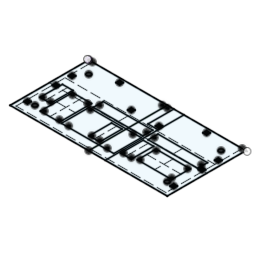
_Drill Guide.1d35a3b7-5dbf-4833-a90d-6280b39ef4eb (Autodesk Fusion 360 design; units mm, degrees)
Autodesk Fusion 360 part; units mm, degrees
sketch "Sketch1" plane through (0, 0, 0) normal (0, 1, 0) x (1, 0, 0)
  line L0 (0, 0) -> (304.8, 0) construction
  line L1 (304.8, 0) -> (304.8, -152.4) construction
  line L2 (304.8, -152.4) -> (0, -152.4) construction
  line L3 (0, -152.4) -> (0, 0) construction
  line L4 (297.775, 0) -> (297.775, -147.9) construction
  line L5 (297.775, -147.9) -> (7.025, -147.9) construction
  line L6 (7.025, -147.9) -> (7.025, 0) construction
  line L7 (39.025, -70.5) -> (76.025, -70.5)
  line L8 (76.025, -70.5) -> (76.025, -132.9)
  line L9 (76.025, -132.9) -> (39.025, -132.9)
  line L10 (39.025, -132.9) -> (39.025, -70.5)
  circle A0 centre (42.95, -74.425) radius 1.625
  line L11 (57.525, -70.5) -> (57.525, -132.9) construction
  circle A1 centre (72.1, -74.425) radius 1.625
  line L12 (39.025, -101.7) -> (76.025, -101.7) construction
  circle A2 centre (72.1, -128.975) radius 1.625
  circle A3 centre (42.95, -128.975) radius 1.625
  line L13 (15.525, -66.5) -> (35.875, -66.5)
  line L14 (35.875, -66.5) -> (35.875, -109.9)
  line L15 (35.875, -109.9) -> (15.525, -109.9)
  line L16 (15.525, -109.9) -> (15.525, -66.5)
  circle A4 centre (18.08, -107.345) radius 1.555
  line L17 (25.7, -66.5) -> (25.7, -109.9) construction
  circle A5 centre (33.32, -107.345) radius 1.555
  line L18 (80.025, -79.56) -> (181.625, -79.56)
  line L19 (181.625, -79.56) -> (181.625, -132.9)
  line L20 (181.625, -132.9) -> (80.025, -132.9)
  line L21 (80.025, -132.9) -> (80.025, -79.56)
  circle A6 centre (85.105, -82.1) radius 1.65
  circle A7 centre (91.455, -130.36) radius 1.65
  circle A8 centre (167.655, -82.1) radius 1.65
  circle A9 centre (166.385, -130.36) radius 1.65
  line L22 (7.025, -52.9) -> (297.775, -52.9) construction
  line L23 (187.625, -82) -> (207.975, -82)
  line L24 (207.975, -82) -> (207.975, -125.4)
  line L25 (207.975, -125.4) -> (187.625, -125.4)
  line L26 (187.625, -125.4) -> (187.625, -82)
  circle A10 centre (190.18, -122.845) radius 1.555
  line L27 (197.8, -82) -> (197.8, -125.4) construction
  circle A11 centre (205.42, -122.845) radius 1.555
  circle A12 centre (145.82, -124.545) radius 1.555
  circle A13 centre (130.58, -124.545) radius 1.555
  line L28 (148.375, -83.7) -> (148.375, -127.1)
  line L29 (148.375, -127.1) -> (128.025, -127.1)
  line L30 (128.025, -127.1) -> (128.025, -83.7)
  line L31 (138.2, -83.7) -> (138.2, -127.1) construction
  line L32 (128.025, -83.7) -> (148.375, -83.7)
  line L33 (215.125, -84.4) -> (281.275, -84.4)
  line L34 (281.275, -84.4) -> (281.275, -120.4)
  line L35 (281.275, -120.4) -> (215.125, -120.4)
  line L36 (215.125, -120.4) -> (215.125, -84.4)
  circle A14 centre (217.675, -86.95) radius 1.55
  line L37 (248.2, -84.4) -> (248.2, -120.4) construction
  line L38 (215.125, -102.4) -> (281.275, -102.4) construction
  circle A15 centre (278.725, -86.95) radius 1.55
  circle A16 centre (217.675, -117.85) radius 1.55
  circle A17 centre (278.725, -117.85) radius 1.55
  line L39 (84.065, -55.86) -> (180.125, -55.86)
  line L40 (180.125, -55.86) -> (180.125, -74.96)
  line L41 (180.125, -74.96) -> (84.065, -74.96)
  line L42 (84.065, -74.96) -> (84.065, -55.86)
  circle A18 centre (177.625, -65.46) radius 1.5
  line L43 (132.095, -55.86) -> (132.095, -74.96) construction
  circle A19 centre (86.565, -65.46) radius 1.5
  line L44 (191.715, -76.4) -> (191.715, -57.3)
  line L45 (239.745, -57.3) -> (239.745, -76.4) construction
  line L46 (287.775, -76.4) -> (191.715, -76.4)
  line L47 (191.715, -57.3) -> (287.775, -57.3)
  circle A20 centre (285.275, -66.9) radius 1.5
  circle A21 centre (194.215, -66.9) radius 1.5
  line L48 (287.775, -57.3) -> (287.775, -76.4)
  line L49 (7.025, -125.9) -> (14.025, -125.9)
  line L50 (14.025, -125.9) -> (14.025, -132.9)
  line L51 (14.025, -132.9) -> (7.025, -132.9)
  line L52 (7.025, -132.9) -> (7.025, -125.9)
  line L53 (7.025, -70.9) -> (14.025, -70.9)
  line L54 (14.025, -70.9) -> (14.025, -77.9)
  line L55 (14.025, -77.9) -> (7.025, -77.9)
  line L56 (7.025, -77.9) -> (7.025, -70.9)
  line L57 (7.025, -39.4) -> (14.025, -39.4)
  line L58 (14.025, -39.4) -> (14.025, -46.4)
  line L59 (14.025, -46.4) -> (7.025, -46.4)
  line L60 (7.025, -46.4) -> (7.025, -39.4)
  line L61 (122.025, -39.4) -> (129.025, -39.4)
  line L62 (129.025, -39.4) -> (129.025, -46.4)
  line L63 (129.025, -46.4) -> (122.025, -46.4)
  line L64 (122.025, -46.4) -> (122.025, -39.4)
  line L65 (152.4, 0) -> (152.4, -147.9) construction
  circle A22 centre (68.025, -8) radius 1.5
  circle A23 centre (10.525, -42.9) radius 1.5
  circle A24 centre (10.525, -74.4) radius 1.5
  circle A25 centre (10.525, -129.4) radius 1.5
  circle A26 centre (125.525, -42.9) radius 1.5
  line L66 (0, 0) -> (304.8, 0)
  line L67 (304.8, 0) -> (304.8, -152.4)
  line L68 (304.8, -152.4) -> (0, -152.4)
  line L69 (0, -152.4) -> (0, 0)
  line L70 (152.4, 0) -> (152.4, -152.4)
  line L71 (-0.1, 0) -> (-2.5, 0)
  line L72 (307.3, 0) -> (304.9, 0)
  line L73 (0, 0) -> (-0.1, 0)
  line L74 (304.9, 0) -> (304.8, 0)
  line L75 (184.625, 0) -> (184.625, -152.4)
  line L76 (165, 0) -> (165, -50)
  line L77 (165, -50) -> (184.625, -50)
  circle A27 centre (24, -128.4) radius 3.95
  line L78 (0, -76.2) -> (304.8, -76.2) construction
  circle A28 centre (24, -24) radius 3.95
  circle A29 centre (280.8, -24) radius 3.95
  circle A30 centre (280.8, -128.4) radius 3.95
  circle A31 centre (147.4, -4.75) radius 1.5
  circle A32 centre (157.4, -4.75) radius 1.5
  line L79 (64.525, -4.5) -> (71.525, -4.5)
  line L80 (71.525, -4.5) -> (71.525, -11.5)
  line L81 (71.525, -11.5) -> (64.525, -11.5)
  line L82 (64.525, -11.5) -> (64.525, -4.5)
  line L83 (233.275, -11.5) -> (240.275, -11.5)
  circle A33 centre (236.775, -8) radius 1.5
  line L84 (240.275, -11.5) -> (240.275, -4.5)
  line L85 (240.275, -4.5) -> (233.275, -4.5)
  line L86 (233.275, -4.5) -> (233.275, -11.5)
  line L87 (297.775, -39.4) -> (290.775, -39.4)
  line L88 (290.775, -39.4) -> (290.775, -46.4)
  circle A34 centre (294.275, -42.9) radius 1.5
  line L89 (290.775, -46.4) -> (297.775, -46.4)
  line L90 (297.775, -46.4) -> (297.775, -39.4)
  line L91 (297.775, -70.9) -> (290.775, -70.9)
  line L92 (290.775, -70.9) -> (290.775, -77.9)
  circle A35 centre (294.275, -74.4) radius 1.5
  line L93 (297.775, -77.9) -> (297.775, -70.9)
  line L94 (290.775, -77.9) -> (297.775, -77.9)
  line L95 (297.775, -125.9) -> (290.775, -125.9)
  line L96 (290.775, -125.9) -> (290.775, -132.9)
  circle A36 centre (294.275, -129.4) radius 1.5
  line L97 (290.775, -132.9) -> (297.775, -132.9)
  line L98 (297.775, -132.9) -> (297.775, -125.9)
  circle A37 centre (179.275, -42.9) radius 1.5
  line L99 (175.775, -46.4) -> (182.775, -46.4)
  line L100 (182.775, -46.4) -> (182.775, -39.4)
  line L101 (175.775, -39.4) -> (175.775, -46.4)
  line L102 (182.775, -39.4) -> (175.775, -39.4)
  dimension "d1" = 304.8
  dimension "d2" = 152.4
  dimension "d3" = 290.75
  dimension "d4" = 147.9
  dimension "d5" = 7.025
  dimension "d6" = 3.25
  dimension "d7" = 37
  dimension "d8" = 62.4
  dimension "d9" = 3.925
  dimension "d10" = 3.925
  dimension "d11" = 32
  dimension "d13" = 20.35
  dimension "d14" = 43.4
  dimension "d15" = 3.11
  dimension "d16" = 2.555
  dimension "d17" = 2.555
  dimension "d18" = 8.5
  dimension "d19" = 42.5
  dimension "d20" = 19.5
  dimension "d21" = 101.6
  dimension "d22" = 53.34
  dimension "d23" = 3.3
  dimension "d24" = 3.3
  dimension "d25" = 3.3
  dimension "d26" = 3.3
  dimension "d27" = 96.52
  dimension "d28" = 2.54
  dimension "d29" = 13.97
  dimension "d30" = 2.54
  dimension "d31" = 15.24
  dimension "d32" = 50.8
  dimension "d33" = 90.17
  dimension "d34" = 50.8
  dimension "d35" = 19.5
  dimension "d36" = 73
  dimension "d38" = 20.35
  dimension "d39" = 43.4
  dimension "d40" = 3.11
  dimension "d41" = 2.555
  dimension "d42" = 2.555
  dimension "d43" = 27
  dimension "d45" = 6
  dimension "d46" = 20.35
  dimension "d47" = 43.4
  dimension "d48" = 3.11
  dimension "d49" = 2.555
  dimension "d50" = 2.555
  dimension "d51" = 25.3
  dimension "d52" = 48
  dimension "d53" = 66.15
  dimension "d54" = 36
  dimension "d55" = 3.1
  dimension "d56" = 2.55
  dimension "d57" = 2.55
  dimension "d58" = 32
  dimension "d59" = 16.5
  dimension "d60" = 96.06
  dimension "d61" = 19.1
  dimension "d62" = 3
  dimension "d63" = 9.6
  dimension "d64" = 2.5
  dimension "d65" = 4.6
  dimension "d66" = 1.5
  dimension "d67" = 96.06
  dimension "d68" = 19.1
  dimension "d69" = 3
  dimension "d70" = 9.6
  dimension "d71" = 2.5
  dimension "d72" = 10
  dimension "d73" = 8
  dimension "d74" = 7
  dimension "d75" = 7
  dimension "d76" = 15
  dimension "d77" = 7
  dimension "d78" = 7
  dimension "d79" = 70
  dimension "d80" = 7
  dimension "d81" = 7
  dimension "d82" = 101.5
  dimension "d86" = 7
  dimension "d87" = 7
  dimension "d88" = 115
  dimension "d89" = 101.5
  dimension "d90" = 3
  dimension "d93" = 3
  dimension "d94" = 3.5
  dimension "d95" = 3.5
  dimension "d96" = 3
  dimension "d97" = 3.5
  dimension "d98" = 3.5
  dimension "d99" = 3
  dimension "d100" = 3.5
  dimension "d101" = 3.5
  dimension "d102" = 3
  dimension "d103" = 3.5
  dimension "d104" = 3.5
  dimension "d127" = 3
  dimension "d130" = 19.625
  dimension "d131" = 50
  dimension "d132" = 7.9
  dimension "d133" = 24
  dimension "d134" = 24
  dimension "d135" = 3
  dimension "d136" = 3
  dimension "d137" = 10
  dimension "d140" = 5
  dimension "d141" = 4.75
  dimension "d145" = 7
  dimension "d146" = 7
  dimension "d147" = 3.5
  dimension "d148" = 3.5
  dimension "d149" = 4.5
  dimension "d150" = 4.75
  dimension "d151" = 57.5
  dimension "d152" = 52.9
  constraint horizontal L0
  constraint vertical L1
  constraint horizontal L2
  constraint vertical L3
  constraint coincident L0.start L3.end
  constraint vertical L4
  constraint horizontal L5
  constraint vertical L6
  constraint coincident L0 L6.end
  constraint horizontal L7
  constraint vertical L8
  constraint horizontal L9
  constraint vertical L10
  constraint midpoint L7 L11.start
  constraint midpoint L9 L11.end
  constraint symmetric A0 L11 A1
  constraint midpoint L10 L12.start
  constraint midpoint L8 L12.end
  constraint symmetric A0 L12 A3
  constraint symmetric A1 L12 A2
  constraint horizontal L13
  constraint vertical L14
  constraint horizontal L15
  constraint vertical L16
  constraint midpoint L13 L17.start
  constraint midpoint L15 L17.end
  constraint symmetric A4 L17 A5
  constraint horizontal L18
  constraint vertical L19
  constraint horizontal L20
  constraint vertical L21
  constraint coincident L6 L22.start
  constraint coincident L4 L22.end
  constraint perpendicular L4 L22
  constraint horizontal L23
  constraint vertical L24
  constraint horizontal L25
  constraint vertical L26
  constraint midpoint L23 L27.start
  constraint midpoint L25 L27.end
  constraint symmetric A10 L27 A11
  constraint horizontal L32
  constraint vertical L28
  constraint horizontal L29
  constraint vertical L30
  constraint midpoint L31.start L32
  constraint midpoint L31.end L29
  constraint symmetric A12 A13 L31
  constraint horizontal L33
  constraint vertical L34
  constraint horizontal L35
  constraint vertical L36
  constraint midpoint L33 L37.start
  constraint midpoint L35 L37.end
  constraint midpoint L36 L38.start
  constraint midpoint L34 L38.end
  constraint symmetric A14 L37 A15
  constraint symmetric A14 L38 A16
  constraint symmetric L38 A15 A17
  constraint horizontal L39
  constraint vertical L40
  constraint horizontal L41
  constraint vertical L42
  constraint midpoint L39 L43.start
  constraint midpoint L41 L43.end
  constraint symmetric A18 L43 A19
  constraint horizontal L47
  constraint vertical L48
  constraint horizontal L46
  constraint vertical L44
  constraint midpoint L45.start L47
  constraint midpoint L45.end L46
  constraint symmetric L45 A20 A21
  constraint horizontal L49
  constraint vertical L50
  constraint horizontal L51
  constraint vertical L52
  constraint coincident L6 L49.start
  constraint horizontal L53
  constraint vertical L54
  constraint horizontal L55
  constraint vertical L56
  constraint coincident L6 L53.start
  constraint horizontal L57
  constraint vertical L58
  constraint horizontal L59
  constraint vertical L60
  constraint coincident L6 L57.start
  constraint horizontal L61
  constraint vertical L62
  constraint horizontal L63
  constraint vertical L64
  constraint midpoint L5 L65.end
  constraint horizontal L66
  constraint vertical L67
  constraint horizontal L68
  constraint vertical L69
  constraint midpoint L68 L70.end
  constraint perpendicular L1 L72
  constraint perpendicular L67 L74
  constraint coincident L66 L75.start
  constraint coincident L68 L75.end
  constraint perpendicular L68 L75
  constraint coincident L66 L76.start
  constraint perpendicular L22 L76
  constraint coincident L75 L77.end
  constraint perpendicular L75 L77
  constraint midpoint L3 L78.start
  constraint midpoint L67 L78.end
  constraint symmetric A27 L78 A28
  constraint symmetric L70 A27 A30
  constraint symmetric L70 A28 A29
  constraint horizontal L79
  constraint vertical L80
  constraint horizontal L81
  constraint vertical L82
  constraint symmetric L49.start L65 L95.start
  constraint symmetric L49.end L65 L95.end
  constraint symmetric L50.end L65 L96.end
  constraint symmetric L51.end L65 L97.end
  constraint symmetric L53.start L65 L91.start
  constraint symmetric L53.end L65 L91.end
  constraint symmetric L54.end L65 L92.end
  constraint symmetric L55.end L65 L93.start
  constraint symmetric L57.start L65 L87.start
  constraint symmetric L57.end L65 L87.end
  constraint symmetric L58.end L65 L88.end
  constraint symmetric L59.end L65 L89.end
  constraint symmetric L61.start L65 L100.end
  constraint symmetric L61.end L65 L101.start
  constraint symmetric L62.end L65 L99.start
  constraint symmetric L63.end L65 L99.end
  constraint symmetric L65 A22 A33
  constraint symmetric L65 A23 A34
  constraint symmetric L65 A24 A35
  constraint symmetric L65 A25 A36
  constraint symmetric L65 A26 A37
  constraint symmetric L65 L79.start L84.end
  constraint symmetric L65 L79.end L85.end
  constraint symmetric L65 L80.end L83.start
  constraint symmetric L65 L81.end L83.end
  measures "d1" distance of L1.end L2.end
  measures "d2" distance of L0.end L1.end
  measures "d3" distance of L6.end L4.start
  measures "d4" distance of L6.end L5.end
  measures "d5" distance of L3 L6
  measures "d6" diameter of A0
  measures "d7" distance of L7.start L7.end
  measures "d8" distance of L7.end L8.end
  measures "d9" distance of L7 A0.centre
  measures "d10" distance of L10 A0.centre
  measures "d11" distance of L6 L10
  measures "d13" distance of L13.start L13.end
  measures "d14" distance of L13.start L15.end
  measures "d15" diameter of A4
  measures "d16" distance of L16 A4.centre
  measures "d17" distance of L15 A4.centre
  measures "d18" distance of L6 L16
  measures "d19" distance of L2 L15
  measures "d20" distance of L2 L9
  measures "d21" distance of L18.start L18.end
  measures "d22" distance of L18.start L20.end
  measures "d23" diameter of A6
  measures "d24" diameter of A7
  measures "d25" diameter of A8
  measures "d26" diameter of A9
  measures "d27" distance of L19 A6.centre
  measures "d28" distance of L18 A6.centre
  measures "d29" distance of L19 A8.centre
  measures "d30" distance of L18 A8.centre
  measures "d31" distance of L19 A9.centre
  measures "d32" distance of L18 A9.centre
  measures "d33" distance of L19 A7.centre
  measures "d34" distance of L18 A7.centre
  measures "d35" distance of L2 L20
  measures "d36" distance of L6 L21
  measures "d38" distance of L23.start L23.end
  measures "d39" distance of L23.start L25.end
  measures "d40" diameter of A10
  measures "d41" distance of A10.centre L26
  measures "d42" distance of A10.centre L25
  measures "d43" distance of L2 L25
  measures "d45" distance of L19 L26
  measures "d46" distance of L30.end L28.start
  measures "d47" distance of L30.end L29.end
  measures "d48" diameter of A13
  measures "d49" distance of A13.centre L30
  measures "d50" distance of A13.centre L29
  measures "d51" distance of L2 L29
  measures "d52" distance of L21 L30
  measures "d53" distance of L33.start L33.end
  measures "d54" distance of L33.start L35.end
  measures "d55" diameter of A14
  measures "d56" distance of L33 A14.centre
  measures "d57" distance of L36 A14.centre
  measures "d58" distance of L2 L35
  measures "d59" distance of L4 L34
  measures "d60" distance of L39.start L39.end
  measures "d61" distance of L39.start L41.end
  measures "d62" diameter of A18
  measures "d63" distance of L39 A18.centre
  measures "d64" distance of L40 A18.centre
  measures "d65" distance of L18 L41
  measures "d66" distance of L19 L40
  measures "d67" distance of L44.end L47.end
  measures "d68" distance of L44.end L44.start
  measures "d69" diameter of A20
  measures "d70" distance of A20.centre L47
  measures "d71" distance of A20.centre L48
  measures "d72" distance of L4 L48
  measures "d73" distance of L33 L46
  measures "d74" distance of L49.start L49.end
  measures "d75" distance of L49.start L51.end
  measures "d76" distance of L5 L51
  measures "d77" distance of L53.start L53.end
  measures "d78" distance of L53.start L55.end
  measures "d79" distance of L5 L55
  measures "d80" distance of L57.start L57.end
  measures "d81" distance of L57.start L59.end
  measures "d82" distance of L5 L59
  measures "d86" distance of L61.start L63.end
  measures "d87" distance of L62.end L63.end
  measures "d88" distance of L6 L64
  measures "d89" distance of L5 L63
  measures "d90" diameter of A22
  measures "d93" diameter of A23
  measures "d94" distance of L58 A23.centre
  measures "d95" distance of L57 A23.centre
  measures "d96" diameter of A24
  measures "d97" distance of L53 A24.centre
  measures "d98" distance of L54 A24.centre
  measures "d99" diameter of A25
  measures "d100" distance of L50 A25.centre
  measures "d101" distance of L49 A25.centre
  measures "d102" diameter of A26
  measures "d103" distance of L62 A26.centre
  measures "d104" distance of L61 A26.centre
  measures "d127" distance of L26 L75
  measures "d130" distance of L75 L76
  measures "d131" distance of L66 L77
  measures "d132" diameter of A27
  measures "d133" distance of L69 A27.centre
  measures "d134" distance of L68 A27.centre
  measures "d135" diameter of A31
  measures "d136" diameter of A32
  measures "d137" distance of A31.centre A32.centre
  measures "d140" distance of L70 A31.centre
  measures "d141" distance of L0 A32.centre
  measures "d145" distance of L79.start L79.end
  measures "d146" distance of L79.start L81.end
  measures "d147" distance of A22.centre L82
  measures "d148" distance of A22.centre L79
  measures "d149" distance of L0 L79
  measures "d150" distance of L66 A31.centre
  measures "d151" distance of L6 L82
  measures "d152" distance of L0 L22
extrude "Extrude7" add sketch "Sketch1" along normal blind 1 contours L7 L8 L9 L10 | L13 L14 L15 L16 | L18 L20 L21 L39 L41 L42 L66 L68 L69 L70 | L18 L20 L21 L70 | L18 L19 L20 L39 L40 L41 L66 L68 L70 L75 L76 L77 | L18 L19 L20 L70 | L39 L40 L41 L70 | L39 L41 L42 L70 | L28 L29 L30 L32 | L49 L50 L51 L52 | L53 L54 L55 L56 | L57 L58 L59 L60 | L61 L62 L63 L64 | L79 L80 L81 L82
equation "d3 = 297.75 mm - ( 3.5 * 2 ) * 1 mm"
equation "d5 = ( d1 - d3 ) / 2"
equation "d9 = d6 / 2 + 2.3 mm"
equation "d10 = d9"
equation "d16 = d15 / 2 + 1 mm"
equation "d17 = d16"
equation "d24 = d23"
equation "d25 = d23"
equation "d26 = d23"
equation "d30 = d28"
equation "d34 = d32"
equation "d41 = d15 / 2 + 1 mm"
equation "d42 = d16"
equation "d49 = d15 / 2 + 1 mm"
equation "d50 = d16"
equation "d56 = d55 / 2 + 1 mm"
equation "d57 = d55 / 2 + 1 mm"
equation "d63 = d62 / 2 + 8.1 mm"
equation "d64 = d62 / 2 + 1 mm"
equation "d70 = d62 / 2 + 8.1 mm"
equation "d71 = d62 / 2 + 1 mm"
equation "d94 = d80 / 2"
equation "d95 = d81 / 2"
equation "d97 = d78 / 2"
equation "d98 = d77 / 2"
equation "d100 = d74 / 2"
equation "d101 = d75 / 2"
equation "d103 = d87 / 2"
equation "d104 = d86 / 2"
equation "d140 = d137 / 2"
equation "d147 = d145 / 2"
equation "d148 = d146 / 2"
